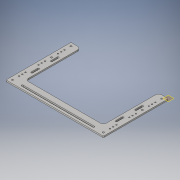
# Autodesk Inventor part: vrRig_v08p1_base
Saved by Autodesk Inventor 2016 (Build 200138000, 138)
## iProperties
Created: 2018-01-13
Part Number: vrRig_v08p1_base
Material: Generic
Document SubType Name: Modeling
Designer: harveylab
Density: 1 g/cm^3
Appearance: Default
Author: harveylab
Autodesk Inventor part; units mm, degrees
ref_plane "YZ Plane" through (0, 0, 0) normal (1, 0, 0) x (0, 1, 0)
ref_plane "XZ Plane" through (0, 0, 0) normal (0, 1, 0) x (-1, 0, 0)
ref_plane "XY Plane" through (0, 0, 0) normal (0, 0, 1) x (1, 0, 0)
sketch "Sketch1" plane through (0, 0, 0) normal (0, 1, 0) x (-1, 0, 0)
  circle A0 centre (368.3, 203.2) radius 2.54 construction
  circle A1 centre (368.3, 241.3) radius 3.302
  circle A2 centre (368.3, 127) radius 2.54 construction
  circle A3 centre (368.3, 88.9) radius 3.302
  circle A4 centre (368.3, 50.8) radius 2.54 construction
  circle A5 centre (368.3, 12.7) radius 3.302
  line L0 (190.5, 244.602) -> (330.2, 244.602)
  line L1 (330.2, 244.602) -> (190.5, 244.602)
  arc A6 (330.2, 237.998) -> (330.2, 244.602) centre (330.2, 241.3) ccw
  line L2 (190.5, 237.998) -> (330.2, 237.998)
  line L3 (381, 251.46) -> (381, 2.54)
  line L4 (378.46, 0) -> (355.6, 0)
  line L5 (355.6, 0) -> (355.6, 0)
  circle A7 centre (368.3, 38.1) radius 2.54 construction
  circle A8 centre (368.3, 63.5) radius 2.54 construction
  circle A9 centre (368.3, 127) radius 2.54 construction
  circle A10 centre (368.3, 114.3) radius 2.54 construction
  circle A11 centre (368.3, 139.7) radius 2.54 construction
  circle A12 centre (368.3, 203.2) radius 2.54 construction
  circle A13 centre (368.3, 190.5) radius 2.54 construction
  circle A14 centre (368.3, 215.9) radius 2.54 construction
  line L6 (355.6, 0) -> (355.6, 25.4) construction
  line L7 (355.6, 25.4) -> (381, 25.4) construction
  line L8 (368.3, 88.9) -> (355.6, 88.9) construction
  arc A15 (352.298, 76.2) -> (358.902, 76.2) centre (355.6, 76.2) ccw
  arc A16 (358.902, 101.6) -> (352.298, 101.6) centre (355.6, 101.6) ccw
  line L9 (358.902, 76.2) -> (358.902, 101.6)
  line L10 (352.298, 101.6) -> (352.298, 76.2)
  line L11 (368.3, 139.7) -> (368.3, 165.1) construction
  line L12 (368.3, 165.1) -> (355.6, 165.1) construction
  arc A17 (352.298, 152.4) -> (358.902, 152.4) centre (355.6, 152.4) ccw
  arc A18 (358.902, 177.8) -> (352.298, 177.8) centre (355.6, 177.8) ccw
  line L13 (358.902, 152.4) -> (358.902, 177.8)
  line L14 (352.298, 177.8) -> (352.298, 152.4)
  arc A19 (342.9, 12.7) -> (355.6, 0) centre (355.6, 12.7) ccw
  line L15 (378.46, 254) -> (190.5, 254)
  arc A20 (378.46, 0) -> (381, 2.54) centre (378.46, 2.54) ccw
  arc A21 (381, 251.46) -> (378.46, 254) centre (378.46, 251.46) ccw
  line L16 (190.5, 228.6) -> (190.5, 159.7209) construction
  line L17 (330.2, 215.9) -> (190.5, 215.9)
  line L18 (342.9, 12.7) -> (342.9, 203.2)
  arc A22 (342.9, 203.2) -> (330.2, 215.9) centre (330.2, 203.2) ccw
  circle A23 centre (12.7, 203.2) radius 2.54 construction
  circle A24 centre (12.7, 241.3) radius 3.302
  circle A25 centre (12.7, 127) radius 2.54 construction
  circle A26 centre (12.7, 88.9) radius 3.302
  circle A27 centre (12.7, 50.8) radius 2.54 construction
  circle A28 centre (12.7, 12.7) radius 3.302
  line L19 (190.5, 244.602) -> (50.8, 244.602)
  line L20 (50.8, 244.602) -> (190.5, 244.602)
  arc A29 (50.8, 244.602) -> (50.8, 237.998) centre (50.8, 241.3) ccw
  line L21 (190.5, 237.998) -> (50.8, 237.998)
  line L22 (0, 251.46) -> (0, 2.54)
  line L23 (2.54, 0) -> (25.4, 0)
  line L24 (25.4, 0) -> (25.4, 0)
  circle A30 centre (12.7, 38.1) radius 2.54 construction
  circle A31 centre (12.7, 63.5) radius 2.54 construction
  circle A32 centre (12.7, 139.7) radius 2.54 construction
  circle A33 centre (12.7, 127) radius 2.54 construction
  circle A34 centre (12.7, 114.3) radius 2.54 construction
  circle A35 centre (12.7, 215.9) radius 2.54 construction
  circle A36 centre (12.7, 203.2) radius 2.54 construction
  circle A37 centre (12.7, 190.5) radius 2.54 construction
  line L25 (25.4, 0) -> (25.4, 25.4) construction
  line L26 (25.4, 25.4) -> (0, 25.4) construction
  line L27 (12.7, 88.9) -> (25.4, 88.9) construction
  arc A38 (22.098, 76.2) -> (28.702, 76.2) centre (25.4, 76.2) ccw
  arc A39 (28.702, 101.6) -> (22.098, 101.6) centre (25.4, 101.6) ccw
  line L28 (22.098, 76.2) -> (22.098, 101.6)
  line L29 (28.702, 101.6) -> (28.702, 76.2)
  line L30 (12.7, 139.7) -> (12.7, 165.1) construction
  line L31 (12.7, 165.1) -> (25.4, 165.1) construction
  line L32 (22.098, 152.4) -> (22.098, 177.8)
  arc A40 (22.098, 152.4) -> (28.702, 152.4) centre (25.4, 152.4) ccw
  line L33 (28.702, 177.8) -> (28.702, 152.4)
  arc A41 (28.702, 177.8) -> (22.098, 177.8) centre (25.4, 177.8) ccw
  arc A42 (25.4, 0) -> (38.1, 12.7) centre (25.4, 12.7) ccw
  line L34 (2.54, 254) -> (190.5, 254)
  arc A43 (0, 2.54) -> (2.54, 0) centre (2.54, 2.54) ccw
  arc A44 (2.54, 254) -> (0, 251.46) centre (2.54, 251.46) ccw
  line L35 (50.8, 215.9) -> (190.5, 215.9)
  line L36 (38.1, 12.7) -> (38.1, 203.2)
  arc A45 (50.8, 215.9) -> (38.1, 203.2) centre (50.8, 203.2) ccw
  point P0 (381, 254)
  point P1 (381, 0)
  point P2 (342.9, 0)
  point P3 (342.9, 228.6)
  point P4 (0, 254)
  point P5 (0, 0)
  point P6 (38.1, 0)
  point P7 (38.1, 228.6)
  dimension "d2" = 12.7
  dimension "d3" = 228.6
  dimension "d6" = 25.4
  dimension "d7" = 25.4
  dimension "d8" = 12.7
  dimension "d10" = 25.4
  dimension "d12" = 12.7
  dimension "d17" = 12.7
  constraints: 74 end point, 52 symmetric about line, 46 centre point, 36 point on circle, 11 point on line, 11 tangent, 3 horizontal, 3 vertical, 2 perpendicular, 1 equal radius, 23 other
  measures "d2" distance of L4.end point (342.9, 0)
  measures "d3" distance of point (342.9, 0) point (342.9, 228.6)
  measures "d6" distance of L6.end L7.end
  measures "d7" distance of L6.start L6.end
  measures "d8" distance of L8.start L8.end
  measures "d10" distance of L11.start L11.end
  measures "d12" radius of A19
  measures "d17" radius of A22
ref_plane "Work Plane1" through (0, 6.35, 0) normal (0, 1, 0) x (1, 0, 0)
extrude "Extrusion4" add sketch "Sketch1" along normal blind 5.588
sketch "Sketch3" plane through (0, 5.588, 0) normal (0, 1, 0) x (1, 0, 0)
  arc A0 (-330.2, -237.998) -> (-330.2, -244.602) centre (-330.2, -241.3) ccw projected
  line L0 (-330.2, -237.998) -> (-50.8, -237.998) projected
  arc A1 (-50.8, -244.602) -> (-50.8, -237.998) centre (-50.8, -241.3) ccw projected
  line L1 (-50.8, -244.602) -> (-330.2, -244.602) projected
  line L2 (-22.098, -76.2) -> (-22.098, -101.6) projected
  arc A2 (-28.702, -101.6) -> (-22.098, -101.6) centre (-25.4, -101.6) ccw projected
  line L3 (-28.702, -101.6) -> (-28.702, -76.2) projected
  arc A3 (-22.098, -76.2) -> (-28.702, -76.2) centre (-25.4, -76.2) ccw projected
  line L4 (-28.702, -177.8) -> (-28.702, -152.4) projected
  arc A4 (-22.098, -152.4) -> (-28.702, -152.4) centre (-25.4, -152.4) ccw projected
  line L5 (-22.098, -152.4) -> (-22.098, -177.8) projected
  arc A5 (-28.702, -177.8) -> (-22.098, -177.8) centre (-25.4, -177.8) ccw projected
  line L6 (-352.298, -152.4) -> (-352.298, -177.8) projected
  arc A6 (-358.902, -177.8) -> (-352.298, -177.8) centre (-355.6, -177.8) ccw projected
  line L7 (-358.902, -177.8) -> (-358.902, -152.4) projected
  arc A7 (-352.298, -152.4) -> (-358.902, -152.4) centre (-355.6, -152.4) ccw projected
  line L8 (-358.902, -101.6) -> (-358.902, -76.2) projected
  arc A8 (-352.298, -76.2) -> (-358.902, -76.2) centre (-355.6, -76.2) ccw projected
  line L9 (-352.298, -76.2) -> (-352.298, -101.6) projected
  arc A9 (-358.902, -101.6) -> (-352.298, -101.6) centre (-355.6, -101.6) ccw projected
  circle A10 centre (-12.7, -88.9) radius 3.302 projected
  circle A11 centre (-12.7, -12.7) radius 3.302 projected
  circle A12 centre (-12.7, -241.3) radius 3.302 projected
  circle A13 centre (-368.3, -12.7) radius 3.302 projected
  circle A14 centre (-368.3, -88.9) radius 3.302 projected
  circle A15 centre (-368.3, -241.3) radius 3.302 projected
  line L10 (-355.6, 0) -> (-378.46, 0) projected
  arc A16 (-378.46, 0) -> (-381, -2.54) centre (-378.46, -2.54) ccw projected
  line L11 (-381, -2.54) -> (-381, -251.46) projected
  arc A17 (-381, -251.46) -> (-378.46, -254) centre (-378.46, -251.46) ccw projected
  line L12 (-378.46, -254) -> (-2.54, -254) projected
  arc A18 (-2.54, -254) -> (0, -251.46) centre (-2.54, -251.46) ccw projected
  line L13 (0, -251.46) -> (0, -2.54) projected
  arc A19 (0, -2.54) -> (-2.54, 0) centre (-2.54, -2.54) ccw projected
  line L14 (-2.54, 0) -> (-25.4, 0) projected
  arc A20 (-25.4, 0) -> (-38.1, -12.7) centre (-25.4, -12.7) ccw projected
  line L15 (-38.1, -12.7) -> (-38.1, -203.2) projected
  arc A21 (-50.8, -215.9) -> (-38.1, -203.2) centre (-50.8, -203.2) ccw projected
  line L16 (-50.8, -215.9) -> (-330.2, -215.9) projected
  arc A22 (-342.9, -203.2) -> (-330.2, -215.9) centre (-330.2, -203.2) ccw projected
  line L17 (-342.9, -203.2) -> (-342.9, -12.7) projected
  arc A23 (-342.9, -12.7) -> (-355.6, 0) centre (-355.6, -12.7) ccw projected
  circle A24 centre (-368.3, -12.7) radius 3.302 projected
  line L18 (-368.3, -12.7) -> (-368.3, -38.1) construction
  line L19 (-368.3, -38.1) -> (-368.3, -50.8) construction
  line L20 (-368.3, -50.8) -> (-368.3, -63.5) construction
  line L21 (-368.3, -88.9) -> (-368.3, -114.3) construction
  line L22 (-368.3, -114.3) -> (-368.3, -127) construction
  line L23 (-368.3, -127) -> (-368.3, -139.7) construction
  line L24 (-368.3, -139.7) -> (-368.3, -165.1) construction
  line L25 (-368.3, -165.1) -> (-368.3, -190.5) construction
  line L26 (-368.3, -190.5) -> (-368.3, -203.2) construction
  line L27 (-368.3, -203.2) -> (-368.3, -215.9) construction
  line L28 (-368.3, -215.9) -> (-368.3, -241.3) construction
  line L29 (-12.7, -12.7) -> (-12.7, -38.1) construction
  line L30 (-12.7, -38.1) -> (-12.7, -50.8) construction
  line L31 (-12.7, -50.8) -> (-12.7, -63.5) construction
  line L32 (-12.7, -88.9) -> (-12.7, -114.3) construction
  line L33 (-12.7, -114.3) -> (-12.7, -127) construction
  line L34 (-12.7, -127) -> (-12.7, -139.7) construction
  line L35 (-12.7, -139.7) -> (-12.7, -165.1) construction
  line L36 (-12.7, -165.1) -> (-12.7, -190.5) construction
  line L37 (-12.7, -190.5) -> (-12.7, -203.2) construction
  line L38 (-12.7, -203.2) -> (-12.7, -215.9) construction
  line L39 (-12.7, -215.9) -> (-12.7, -241.3) construction
  point P0 (0, 0)
  dimension "d22" = 25.4
  dimension "d23" = 12.7
  dimension "d24" = 12.7
  dimension "d25" = 25.4
  dimension "d26" = 12.7
  dimension "d27" = 12.7
  dimension "d28" = 25.4
  dimension "d29" = 25.4
  dimension "d30" = 12.7
  dimension "d31" = 12.7
  dimension "d32" = 25.4
  dimension "d40" = 25.4
  dimension "d41" = 12.7
  dimension "d42" = 12.7
  dimension "d43" = 25.4
  dimension "d44" = 12.7
  dimension "d45" = 12.7
  dimension "d46" = 25.4
  dimension "d47" = 25.4
  dimension "d48" = 12.7
  dimension "d49" = 12.7
  dimension "d50" = 25.4
  constraints: 44 end point, 18 coincident, 12 point on line, 10 vertical
  measures "d22" distance of L18.start L18.end
  measures "d23" distance of L18.end L19.end
  measures "d24" distance of L19.end L20.end
  measures "d25" distance of L21.start L21.end
  measures "d26" distance of L21.end L22.end
  measures "d27" distance of L22.end L23.end
  measures "d28" distance of L24.start L24.end
  measures "d29" distance of L25.start L25.end
  measures "d30" distance of L25.end L26.end
  measures "d31" distance of L26.end L27.end
  measures "d32" distance of L28.start L28.end
  measures "d40" distance of L29.start L30.start
  measures "d41" distance of L30.start L31.start
  measures "d42" distance of L31.start L31.end
  measures "d43" distance of L32.start L32.end
  measures "d44" distance of L32.end L33.end
  measures "d45" distance of L33.end L34.end
  measures "d46" distance of L35.start L35.end
  measures "d47" distance of L36.start L36.end
  measures "d48" distance of L36.end L37.end
  measures "d49" distance of L37.end L38.end
  measures "d50" distance of L39.start L39.end
hole "Hole2" at (-368.3, 5.588, 38.1) at (-368.3, 5.588, 50.8) at (-368.3, 5.588, 63.5) at (-368.3, 5.588, 139.7) at (-368.3, 5.588, 127) at (-368.3, 5.588, 114.3) at (-368.3, 5.588, 215.9) at (-368.3, 5.588, 190.5) at (-368.3, 5.588, 203.2) at (-12.7, 5.588, 139.7) at (-12.7, 5.588, 215.9) at (-12.7, 5.588, 203.2) at (-12.7, 5.588, 190.5) at (-12.7, 5.588, 114.3) at (-12.7, 5.588, 127) at (-12.7, 5.588, 63.5) at (-12.7, 5.588, 50.8) at (-12.7, 5.588, 38.1) direction (0, -1, 0) diameter 4.9784 depth 13.97 tip angle 118 thread size "1/4-20 UNC" class "2B" standard "ANSI Unified Screw Threads"
body "Solid4"
